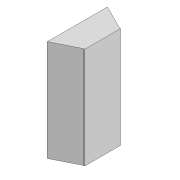
# Autodesk Inventor part: Sliding test wall
Saved by Autodesk Inventor 2020 (Build 240168000, 168)
## iProperties
Created: 2019-11-10
Part Number: Sliding test wall
Material: Generic
Document SubType Name: Modeling
Designer: ball
Density: 1 g/cm^3
Appearance: Default
Author: ball
Autodesk Inventor part; units mm, degrees
ref_plane "YZ Plane" through (0, 0, 0) normal (1, 0, 0) x (0, 1, 0)
ref_plane "XZ Plane" through (0, 0, 0) normal (0, 1, 0) x (-1, 0, 0)
ref_plane "XY Plane" through (0, 0, 0) normal (0, 0, 1) x (1, 0, 0)
sketch "Sketch1" plane through (0, 0, 0) normal (0, 1, 0) x (-1, 0, 0)
  line L0 (0, 4.5) -> (0.254, 4.5)
  line L1 (0.254, -4.5) -> (0, -4.5)
  line L2 (6.35, 4.5) -> (6.35, -4.5)
  line L3 (6.35, 7.548) -> (6.35, 4.5)
  line L4 (6.35, -7.548) -> (6.35, -4.5)
  line L5 (0.254, 4.5) -> (6.35, 7.548)
  line L6 (0.254, -4.5) -> (6.35, -7.548)
  line L7 (0, 4.5) -> (0, -4.5)
  point P0 (0, 0)
  dimension "d16" = 6.096
  dimension "d25" = 9
  dimension "d26" = 3.048
  dimension "d27" = 3.048
  dimension "d28" = 0.254
  dimension "d29" = 0.254
  constraints: 16 end point, 1 horizontal, 1 parallel, 1 point on line, 1 vertical
  measures "d16" distance from line of L4 L1.start
  measures "d25" distance between parallel lines of L0 L1
  measures "d26" vertical distance of L0.end L3.start
  measures "d27" vertical distance of L4.start L1.start
  measures "d28" distance of L1.end L1.start
  measures "d29" distance of L0.start L0.end
extrude "Shape" add sketch "Sketch1" along normal blind 25.4
equation "\"d27\" = d26"
equation "\"d29\" = d28"
body "Solid1"
